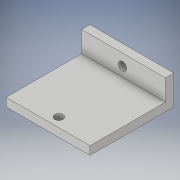
# Autodesk Inventor part: clampforplatform
Saved by Autodesk Inventor 2019 (Build 230136000, 136)
## iProperties
Created: 2020-02-29
Part Number: clampforplatform
Material: Generic
Document SubType Name: Modeling
Designer: Hp
Density: 1 g/cm^3
Appearance: Default
Author: Hp
Autodesk Inventor part; units mm, degrees
ref_plane "YZ Plane" through (0, 0, 0) normal (1, 0, 0) x (0, 1, 0)
ref_plane "XZ Plane" through (0, 0, 0) normal (0, 1, 0) x (-1, 0, 0)
ref_plane "XY Plane" through (0, 0, 0) normal (0, 0, 1) x (1, 0, 0)
sketch "Sketch1" plane through (0, 0, 0) normal (0, 1, 0) x (-1, 0, 0)
  line L0 (10.371, -5.5878) -> (-9.629, -5.5878)
  line L1 (-9.629, -5.5878) -> (-9.629, -25.5878)
  line L2 (-9.629, -25.5878) -> (10.371, -25.5878)
  line L3 (10.371, -25.5878) -> (10.371, -5.5878)
  circle A0 centre (0, -7.8026) radius 1
  point P0 (0, 0)
  dimension "d0" = 20
  dimension "d1" = 20
  dimension "d2" = 2
  constraints: 8 end point, 2 parallel, 1 centre point, 1 horizontal, 1 perpendicular
  measures "d0" distance of L2.end L1.end
  measures "d1" distance of L1.end L0.end
  measures "d2" diameter of A0
extrude "Extrusion1" add sketch "Sketch1" along normal blind 2
sketch "Sketch2" plane through (0, 2, 0) normal (0, 1, 0) x (1, 0, 0)
  line L0 (9.629, 25.5878) -> (-10.371, 25.5878) projected
  line L1 (-10.371, 25.5878) -> (9.629, 25.5878)
  line L2 (9.629, 25.5878) -> (9.629, 23.5878)
  line L3 (9.629, 23.5878) -> (-10.371, 23.5878)
  line L4 (-10.371, 23.5878) -> (-10.371, 25.5878)
  point P0 (0, 0)
  dimension "d5" = 20
  dimension "d6" = 2
  constraints: 8 end point, 2 parallel, 1 horizontal, 1 perpendicular
  measures "d5" distance of L2.end L3.end
  measures "d6" distance of L1.end L2.end
extrude "Extrusion2" add sketch "Sketch2" along normal blind 5
sketch "Sketch3" plane through (-10.371, 2, -23.5878) normal (0, 0, 1) x (1, 0, 0)
  circle A0 centre (9.7422, 2.2933) radius 1
  point P0 (10.371, -2)
  dimension "d9" = 2
  constraints: 1 centre point
  measures "d9" diameter of A0
extrude "Extrusion3" cut sketch "Sketch3" against normal blind 5
body "Solid1"
